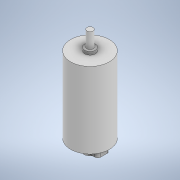
# Autodesk Inventor part: Silnik_SKUA
Saved by Autodesk Inventor 2020 (Build 240168000, 168)
## iProperties
Created: 2019-06-28
Part Number: Silnik_SKUA
Material: Ogólny
Document SubType Name: Modeling
Designer: atmat
Density: 1 g/cm^3
Appearance: Domyślna
Author: atmat
Autodesk Inventor part; units mm, degrees
ref_plane "YZ Plane" through (0, 0, 0) normal (1, 0, 0) x (0, 1, 0)
ref_plane "XZ Plane" through (0, 0, 0) normal (0, 1, 0) x (-1, 0, 0)
ref_plane "XY Plane" through (0, 0, 0) normal (0, 0, 1) x (1, 0, 0)
sketch "Szkic1" plane through (0, 0, 0) normal (0, 1, 0) x (-1, 0, 0)
  circle A0 centre (0, 0) radius 12.5
  dimension "d0" = 25
  constraints: 1 centre point, 1 coincident
  measures "d0" diameter of A0
extrude "Wyciągnięcie proste1" add sketch "Szkic1" along normal blind 56
sketch "Szkic2" plane through (0, 56, 0) normal (0, 1, 0) x (1, 0, 0)
  circle A0 centre (0, 0) radius 2
  dimension "d3" = 4
  constraints: 1 centre point, 1 coincident
  measures "d3" diameter of A0
extrude "Wyciągnięcie proste2" add sketch "Szkic2" along normal blind 12
sketch "Szkic3" plane through (0, 56, 0) normal (0, 1, 0) x (1, 0, 0)
  circle A0 centre (0, 0) radius 3.5
  dimension "d6" = 7
  constraints: 1 centre point, 1 coincident
  measures "d6" diameter of A0
extrude "Wyciągnięcie proste3" add sketch "Szkic3" along normal blind 2
sketch "Szkic4" plane through (0, 0, 0) normal (0, -1, 0) x (1, 0, 0)
  circle A0 centre (0, 0) radius 2 projected
  circle A1 centre (0, 0) radius 4
  circle A2 centre (0, 0) radius 12.5
  dimension "d9" = 8
  constraints: 2 centre point, 2 coincident
  measures "d9" diameter of A1
extrude "Wyciągnięcie proste4" cut sketch "Szkic4" against normal blind 2 contours A2
sketch "Szkic5" plane through (0, 2, 0) normal (0, -1, 0) x (1, 0, 0)
  line L0 (-9, -4) -> (9, -4)
  line L1 (9, -4) -> (9, 4)
  line L2 (9, 4) -> (-9, 4)
  line L3 (-9, 4) -> (-9, -4)
  circle A0 centre (0, 0) radius 4 projected
  circle A1 centre (0, 0) radius 12.5
  dimension "d12" = 9
  dimension "d13" = 18
  constraints: 8 end point, 2 parallel, 2 tangent, 1 centre point, 1 coincident, 1 horizontal, 1 perpendicular
  measures "d12" distance from line of L3 A0.centre
  measures "d13" distance between parallel lines of L1 L3
extrude "Wyciągnięcie proste5" cut sketch "Szkic5" against normal blind 5
fillet "Zaokrąglenie1" radius 2 4 edges at (-9, 4.5, 4) (-9, 4.5, -4) (9, 4.5, 4) (9, 4.5, -4)
